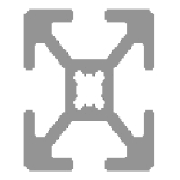
# Autodesk Inventor part: 20-2020
Saved by Autodesk Inventor 2021 (Build 250183000, 183)
## iProperties
Created: 2020-11-08
Part Number: 20-2020
Material: Generic
Document SubType Name: Modeling
Designer: Wes
Manufacturer: 8020
Standards Organization: 8020 Metric
Language: en-US
Size Designation: 20-2020
Categories: <MemberInstance><Categories><Category DisplayName="Structural Shapes" InternalName="089c4875-fa83-4c05-b084-43b9cc11f5ed" Mnemonic="GRDR"><CategoryParameter DisplayName="Mass per Length Unit" InternalName="0bb95a10-148f-4027-a459-38d7b056702a" Mnemonic="shpmass"/><CategoryParameter DisplayName="Section Area" InternalName="1ff91680-64b0-4202-b9a3-7fd3f94bba3b" Mnemonic="secarea"/><CategoryParameter DisplayName="Radius of Gyration (x)" InternalName="25778675-03e9-40c1-b6a8-4a9ed693320d" Mnemonic="gyrradx"/><CategoryParameter DisplayName="Torsional Rigidity Modulus" InternalName="26c1ec35-5026-4c63-ad0a-751cf684a536" Mnemonic="torrigmod"/><CategoryParameter DisplayName="Distance of the Center of Gravity X-X" InternalName="26c9bdb8-9c79-4b4f-a92e-8e197583c9c4" Mnemonic="grcendistX"/><CategoryParameter DisplayName="Legacy Member ID" InternalName="340afe4f-75d7-48d3-ab7d-943f3c3da468" Mnemonic="LegacyMemberID"/><CategoryParameter DisplayName="Base Length" InternalName="42e34263-8f20-4d0e-ad48-bf1385b87c24" Mnemonic="shplen"/><CategoryParameter DisplayName="Moment of Inertia (y)" InternalName="4b9f58ea-bced-460e-81ea-3d29ca5a49e3" Mnemonic="inermomy"/><CategoryParameter DisplayName="Moment of Inertia (x)" InternalName="4cd780bc-73d7-43ac-917a-579e5cbd684d" Mnemonic="inermomx"/><CategoryParameter DisplayName="Custom Base Point" InternalName="4f1d1b73-316d-484b-a3df-9cbabb16eb77" Mnemonic="shpBasePoint"/><CategoryParameter DisplayName="Shape Height" InternalName="50274e7d-5ac0-4796-92cb-c59e54983c67" Mnemonic="shpheig"/><CategoryParameter DisplayName="Section Module (y)" InternalName="59eaa5e9-d227-48dc-b6c1-6920f96e0f95" Mnemonic="secmody"/><CategoryParameter DisplayName="Section Designation" InternalName="5a64d034-428d-49c8-ba32-7619764de20f" Mnemonic="shpdes"/><CategoryParameter DisplayName="Section Module (x)" InternalName="72cfad18-cf51-4ed4-aaa7-c6b224f8419f" Mnemonic="secmodx"/><CategoryParameter DisplayName="Torsional Section Modulus" InternalName="7c55a8dc-8844-49f9-a867-cc677b30ec9a" Mnemonic="torsecmod"/><CategoryParameter DisplayName="Shape Width" InternalName="7c717d54-a18f-4666-b4d4-573cce22c62c" Mnemonic="shpwdth"/><CategoryParameter DisplayName="Second Shape Thickness" InternalName="9251a8e1-85fd-4e47-af99-afdb762317d9" Mnemonic="shpthick2"/><CategoryParameter DisplayName="FG Authored" InternalName="9c666724-f362-4ea7-ac62-f6a007de5c69" Mnemonic="shpFGAuto"/><CategoryParameter DisplayName="Distance of the Center of Gravity Y-Y" InternalName="bcc4fb17-7af4-436a-8f8c-d0aa3b0248c5" Mnemonic="grcendistY"/><CategoryParameter DisplayName="Radius of Gyration (y)" InternalName="bfa18ebe-1636-4dbe-8d42-b263e0b73184" Mnemonic="gyrrady"/><CategoryParameter DisplayName="Shape Thickness" InternalName="d109cf76-8eb4-42fc-9800-4409734adc67" Mnemonic="shpthick"/><CategoryParameter DisplayName="Coefficient of Shear Displacement" InternalName="de4c90c6-aaa8-468f-a335-6737b311b5d3" Mnemonic="shdispc"/><Category DisplayName="Other" InternalName="f02205ff-2390-476f-921c-0b3185f88e84" Mnemonic="OTHSHP"><CategoryParameter DisplayName="Moment of Inertia (y)" InternalName="044c654e-f649-48ac-84cc-650a29ae31ca" Mnemonic="inermomy"/><CategoryParameter DisplayName="Shape Thickness" InternalName="12b1a788-9233-48fd-a933-2df8ff42b15f" Mnemonic="shpthick"/><CategoryParameter DisplayName="Mass per Length Unit" InternalName="2fd289d6-9394-4d2d-97e6-6659d7d4551d" Mnemonic="shpmass"/><CategoryParameter DisplayName="Radius of Gyration (y)" InternalName="743e1dfe-1bba-408b-b985-cf752b207386" Mnemonic="gyrrady"/><CategoryParameter DisplayName="Section Module (y)" InternalName="88b8bff9-a616-4028-93d5-ed4f79680d13" Mnemonic="secmody"/><CategoryParameter DisplayName="Section Area" InternalName="c46ecdf8-b6eb-4db9-8b25-30258930c1e3" Mnemonic="secarea"/><CategoryParameter DisplayName="Section Module (x)" InternalName="cac70804-9d39-43bb-be17-56ea1f39a6c2" Mnemonic="secmodx"/><CategoryParameter DisplayName="Moment of Inertia (x)" InternalName="ec6737bc-264f-43ed-b0bd-f6d410c2718d" Mnemonic="inermomx"/><CategoryParameter DisplayName="Radius of Gyration (x)" InternalName="ee72c61e-565e-4fd6-b448-66e1e1abcb7e" Mnemonic="gyrradx"/><Category DisplayName="8020" InternalName="79851eee-1260-43d5-80eb-d25638456875" Mnemonic="8020"/></Category></Category><Category DisplayName="DataType" InternalName="23b78d0f-2648-40c6-8793-ca6db495c9e8" Mnemonic="DATATYPE"><CategoryParameter DisplayName="DisplayName" InternalName="05415f3d-3907-474b-a020-eb9d644f4cf3" Mnemonic="DISPLAYNAME"/><CategoryParameter DisplayName="Standard" InternalName="0c0a119c-1e12-4c84-803f-101930972f5e" Mnemonic="STANDARD"/><CategoryParameter DisplayName="Description" InternalName="13903e3d-64b1-4950-80da-f627842ea37f" Mnemonic="DESCRIPTION"/><CategoryParameter DisplayName="Designation" InternalName="2675968c-4ce5-49e0-a4f5-552d29089031" Mnemonic="DESIGNATION"/><CategoryParameter DisplayName="Default Row" InternalName="2af9ec52-faaa-4026-b378-f9fa4afca842" Mnemonic="DEFAULTROW"/><CategoryParameter DisplayName="Folder Name" InternalName="3f06958e-8713-4116-9be7-ed6184ecc97b" Mnemonic="FOLDERNAME"/><CategoryParameter DisplayName="Revision Guid" InternalName="45a75005-10b1-4dfc-8d6d-dfe629f0b93c" Mnemonic="REVISIONGUID"/><CategoryParameter DisplayName="FileName" InternalName="8b46a4cc-9585-4fed-90c3-899f57e09a73" Mnemonic="FILENAME"/><CategoryParameter DisplayName="StdsOrg" InternalName="8f5914e1-4693-403f-8ab5-d37768198c9d" Mnemonic="STDSORG"/><CategoryParameter DisplayName="Family Version" InternalName="914462f6-6e19-4b14-ba84-155b9680b1d0" Mnemonic="FAMILYREVISION"/><CategoryParameter DisplayName="Standard Revision" InternalName="91d5a463-65c2-4fde-b823-3b7fea5e8e17" Mnemonic="STANDARDREVISION"/><CategoryParameter DisplayName="Member Revision" InternalName="a65d44b9-392f-4f4f-857b-e4b3d54996fe" Mnemonic="MEMBERREVISION"/><CategoryParameter DisplayName="ClipFormat" InternalName="bc51e27b-3422-4e78-93ef-cec197ddf230" Mnemonic="CLIPFORMAT"/><CategoryParameter DisplayName="Manufacturer" InternalName="cd6c7a72-a28a-4e50-99a9-2c7f4e13e5ad" Mnemonic="MANUFACTURER"/><CategoryParameter DisplayName="InternalName" InternalName="cf1d0246-76d9-4b4a-8305-fa0409afb5c1" Mnemonic="INTERNALNAME"/><CategoryParameter DisplayName="IsMetric" InternalName="e2385c5b-1ea4-4823-96a8-8de651266ec3" Mnemonic="ISMETRIC"/><Category DisplayName="Part" InternalName="c0e0b642-3bcb-4cc8-9e80-f96d35c4afa4" Mnemonic="PART"><CategoryParameter DisplayName="Part Number" InternalName="016b6077-bfbe-49bd-92c9-d8d59c39c941" Mnemonic="PARTNUMBER"/><CategoryParameter DisplayName="Stock Number" InternalName="4dba7c1c-e26c-444e-836c-b08b433409a8" Mnemonic="STOCKNUMBER"/><CategoryParameter DisplayName="Material Key" InternalName="5c9a8adb-dd2b-4535-b97f-0a94a95fe41f" Mnemonic="MATERIALKEY"/><CategoryParameter DisplayName="Material" InternalName="818a152a-d3c3-49ca-80ee-df7d91421b8e" Mnemonic="MATERIAL"/></Category></Category></Categories><FamilyTemplate Id="20-2020"><FamilyTemplateParameters><FamilyTemplateParameter ObjectType="kModelParameterObject" ValueType="xs:double" Id="12" ObjectReferenceKey="Length"/><FamilyTemplateParameter ObjectType="kPartComponentDefinitionObject" ValueType="xs:string" Id="23" SubObjectId="Material"/><FamilyTemplateParameter ObjectType="kPropertyObject" ValueType="xs:string" Id="26" ObjectReferenceKey="{32853F0F-3444-11d1-9E93-0060B03C1CA6}" SubObjectId="5"/><FamilyTemplateParameter ObjectType="kPropertyObject" ValueType="xs:string" Id="27" ObjectReferenceKey="{32853F0F-3444-11d1-9E93-0060B03C1CA6}" SubObjectId="52"/></FamilyTemplateParameters></FamilyTemplate><CategoryParameterMap><ParamToTemplateMap><ParamToTemplate CategoryParameter="//CategoryParameter[@InternalName='cf1d0246-76d9-4b4a-8305-fa0409afb5c1']" ConstantValue="c23acc55-1e46-463f-aee6-b755883656a5"/><ParamToTemplate CategoryParameter="//CategoryParameter[@InternalName='45a75005-10b1-4dfc-8d6d-dfe629f0b93c']" ConstantValue="7ed192ba-9534-4655-9213-06d96e12c78c"/><ParamToTemplate CategoryParameter="//CategoryParameter[@InternalName='3f06958e-8713-4116-9be7-ed6184ecc97b']" ConstantValue="20-2020"/><ParamToTemplate CategoryParameter="//CategoryParameter[@InternalName='8f5914e1-4693-403f-8ab5-d37768198c9d']" ConstantValue="8020 Metric"/><ParamToTemplate CategoryParameter="//CategoryParameter[@InternalName='0c0a119c-1e12-4c84-803f-101930972f5e']" TemplateParameter="18"/><ParamToTemplate CategoryParameter="//CategoryParameter[@InternalName='91d5a463-65c2-4fde-b823-3b7fea5e8e17']" TemplateParameter="19"/><ParamToTemplate CategoryParameter="//CategoryParameter[@InternalName='cd6c7a72-a28a-4e50-99a9-2c7f4e13e5ad']" ConstantValue="8020"/><ParamToTemplate CategoryParameter="//CategoryParameter[@InternalName='13903e3d-64b1-4950-80da-f627842ea37f']" TemplateParameter="22"/><ParamToTemplate CategoryParameter="//CategoryParameter[@InternalName='05415f3d-3907-474b-a020-eb9d644f4cf3']" ConstantValue="20-2020"/><ParamToTemplate CategoryParameter="//CategoryParameter[@InternalName='914462f6-6e19-4b14-ba84-155b9680b1d0']" ConstantValue="11"/><ParamToTemplate CategoryParameter="//CategoryParameter[@InternalName='bc51e27b-3422-4e78-93ef-cec197ddf230']" ConstantValue="CF_INVENTOR.STDPARTS"/><ParamToTemplate CategoryParameter="//CategoryParameter[@InternalName='e2385c5b-1ea4-4823-96a8-8de651266ec3']" ConstantValue="false"/><ParamToTemplate CategoryParameter="//CategoryParameter[@InternalName='2af9ec52-faaa-4026-b378-f9fa4afca842']" ConstantValue="1"/><ParamToTemplate CategoryParameter="//CategoryParameter[@InternalName='9c666724-f362-4ea7-ac62-f6a007de5c69']" ConstantValue="1"/><ParamToTemplate CategoryParameter="//CategoryParameter[@InternalName='8b46a4cc-9585-4fed-90c3-899f57e09a73']" ConstantValue="20-2020"/><ParamToTemplate CategoryParameter="//CategoryParameter[@InternalName='a65d44b9-392f-4f4f-857b-e4b3d54996fe']" ConstantValue="fbe24d84-f0ed-4629-ad88-4417b9aca3a2"/><ParamToTemplate CategoryParameter="//CategoryParameter[@InternalName='a65d44b9-392f-4f4f-857b-e4b3d54996fe']" ConstantValue="fbe24d84-f0ed-4629-ad88-4417b9aca3a2"/><ParamToTemplate CategoryParameter="//CategoryParameter[@InternalName='2675968c-4ce5-49e0-a4f5-552d29089031']" TemplateParameter="27"/><ParamToTemplate CategoryParameter="//CategoryParameter[@InternalName='42e34263-8f20-4d0e-ad48-bf1385b87c24']" TemplateParameter="12"/><ParamToTemplate CategoryParameter="//CategoryParameter[@InternalName='818a152a-d3c3-49ca-80ee-df7d91421b8e']" TemplateParameter="23"/><ParamToTemplate CategoryParameter="//CategoryParameter[@InternalName='016b6077-bfbe-49bd-92c9-d8d59c39c941']" TemplateParameter="26"/></ParamToTemplateMap></CategoryParameterMap></MemberInstance>
Density: 1 g/cm^3
Appearance: Default
IsCustomPart: 1
_CCFamilyDisplayName: 20-2020
_FrameMemberDoc: Frame Member File
_Version: 15.0.0
_GetPNFromCC: 1
Author: Wes
G_L: 32.165 in
G_W: 0.787 in
G_H: 0.787 in
+A867D917-BCFB-4BDE-AF9A-2008976AA419+CUTDETAIL1: Cut Angle 90.00 deg
Autodesk Inventor part; units mm, degrees
ref_plane "YZ Plane" through (0, 0, 0) normal (1, 0, 0) x (0, 1, 0)
ref_plane "XZ Plane" through (0, 0, 0) normal (0, 1, 0) x (-1, 0, 0)
sketch "20-2020" plane through (0, 0, 0) normal (0, 0, 1) x (1, 0, 0)
  arc A0 (19.287, 13.8034) -> (20.6079, 13.434) centre (20.0514, 13.9905) ccw
  line L0 (20.6079, 13.434) -> (20.7875, 13.6136)
  arc A1 (20.7875, 13.6136) -> (20.4182, 14.9345) centre (20.231, 14.1701) ccw
  arc A2 (20.4182, 14.9345) -> (20.4182, 16.5425) centre (18.483, 15.7385) ccw
  arc A3 (20.4182, 16.5425) -> (20.7875, 17.8634) centre (20.231, 17.3069) ccw
  line L1 (20.7875, 17.8634) -> (20.6079, 18.043)
  arc A4 (20.6079, 18.043) -> (19.287, 17.6736) centre (20.0514, 17.4865) ccw
  arc A5 (19.287, 17.6736) -> (17.679, 17.6736) centre (18.483, 15.7385) ccw
  arc A6 (17.679, 17.6736) -> (16.3581, 18.043) centre (16.9146, 17.4865) ccw
  line L2 (16.3581, 18.043) -> (16.1785, 17.8634)
  arc A7 (16.1785, 17.8634) -> (16.5479, 16.5425) centre (16.735, 17.3069) ccw
  arc A8 (16.5479, 16.5425) -> (16.5479, 14.9345) centre (18.483, 15.7385) ccw
  arc A9 (16.5479, 14.9345) -> (16.1785, 13.6136) centre (16.735, 14.1701) ccw
  line L3 (16.1785, 13.6136) -> (16.3581, 13.434)
  arc A10 (16.3581, 13.434) -> (17.679, 13.8034) centre (16.9146, 13.9905) ccw
  arc A11 (17.679, 13.8034) -> (19.287, 13.8034) centre (18.483, 15.7385) ccw
  line L4 (27.491, 18.3685) -> (27.975, 18.3685)
  arc A12 (26.983, 18.8765) -> (27.491, 18.3685) centre (27.491, 18.8765) ccw
  line L5 (26.983, 21.2255) -> (26.983, 18.8765)
  arc A13 (26.983, 21.2255) -> (26.475, 21.7335) centre (26.475, 21.2255) ccw
  line L6 (25.7491, 21.7335) -> (26.475, 21.7335)
  arc A14 (25.7491, 21.7335) -> (25.3899, 21.5847) centre (25.7491, 21.2255) ccw
  line L7 (22.2868, 18.4816) -> (25.3899, 21.5847)
  arc A15 (22.2868, 18.4816) -> (22.138, 18.1224) centre (22.646, 18.1224) ccw
  line L8 (22.138, 13.3546) -> (22.138, 18.1224)
  arc A16 (22.138, 13.3546) -> (22.2868, 12.9954) centre (22.646, 13.3546) ccw
  line L9 (25.3899, 9.8923) -> (22.2868, 12.9954)
  arc A17 (25.3899, 9.8923) -> (25.7491, 9.7435) centre (25.7491, 10.2515) ccw
  line L10 (26.475, 9.7435) -> (25.7491, 9.7435)
  arc A18 (26.475, 9.7435) -> (26.983, 10.2515) centre (26.475, 10.2515) ccw
  line L11 (26.983, 12.6005) -> (26.983, 10.2515)
  arc A19 (27.491, 13.1085) -> (26.983, 12.6005) centre (27.491, 12.6005) ccw
  line L12 (27.975, 13.1085) -> (27.491, 13.1085)
  arc A20 (28.483, 12.6005) -> (27.975, 13.1085) centre (27.975, 12.6005) ccw
  line L13 (28.483, 7.2385) -> (28.483, 12.6005)
  arc A21 (26.983, 5.7385) -> (28.483, 7.2385) centre (26.983, 7.2385) ccw
  line L14 (21.621, 5.7385) -> (26.983, 5.7385)
  arc A22 (21.113, 6.2465) -> (21.621, 5.7385) centre (21.621, 6.2465) ccw
  line L15 (21.113, 6.7305) -> (21.113, 6.2465)
  arc A23 (21.621, 7.2385) -> (21.113, 6.7305) centre (21.621, 6.7305) ccw
  line L16 (23.97, 7.2385) -> (21.621, 7.2385)
  arc A24 (23.97, 7.2385) -> (24.478, 7.7465) centre (23.97, 7.7465) ccw
  line L17 (24.478, 8.4724) -> (24.478, 7.7465)
  arc A25 (24.478, 8.4724) -> (24.3292, 8.8316) centre (23.97, 8.4724) ccw
  line L18 (21.2261, 11.9347) -> (24.3292, 8.8316)
  arc A26 (21.2261, 11.9347) -> (20.8669, 12.0835) centre (20.8669, 11.5755) ccw
  line L19 (16.0991, 12.0835) -> (20.8669, 12.0835)
  arc A27 (16.0991, 12.0835) -> (15.7399, 11.9347) centre (16.0991, 11.5755) ccw
  line L20 (12.6368, 8.8316) -> (15.7399, 11.9347)
  arc A28 (12.6368, 8.8316) -> (12.488, 8.4724) centre (12.996, 8.4724) ccw
  line L21 (12.488, 7.7465) -> (12.488, 8.4724)
  arc A29 (12.488, 7.7465) -> (12.996, 7.2385) centre (12.996, 7.7465) ccw
  line L22 (15.345, 7.2385) -> (12.996, 7.2385)
  arc A30 (15.853, 6.7305) -> (15.345, 7.2385) centre (15.345, 6.7305) ccw
  line L23 (15.853, 6.2465) -> (15.853, 6.7305)
  arc A31 (15.345, 5.7385) -> (15.853, 6.2465) centre (15.345, 6.2465) ccw
  line L24 (9.983, 5.7385) -> (15.345, 5.7385)
  arc A32 (8.483, 7.2385) -> (9.983, 5.7385) centre (9.983, 7.2385) ccw
  line L25 (8.483, 12.6005) -> (8.483, 7.2385)
  arc A33 (8.991, 13.1085) -> (8.483, 12.6005) centre (8.991, 12.6005) ccw
  line L26 (9.475, 13.1085) -> (8.991, 13.1085)
  arc A34 (9.983, 12.6005) -> (9.475, 13.1085) centre (9.475, 12.6005) ccw
  line L27 (9.983, 10.2515) -> (9.983, 12.6005)
  arc A35 (9.983, 10.2515) -> (10.491, 9.7435) centre (10.491, 10.2515) ccw
  line L28 (11.2169, 9.7435) -> (10.491, 9.7435)
  arc A36 (11.2169, 9.7435) -> (11.5761, 9.8923) centre (11.2169, 10.2515) ccw
  line L29 (14.6792, 12.9954) -> (11.5761, 9.8923)
  arc A37 (14.6792, 12.9954) -> (14.828, 13.3546) centre (14.32, 13.3546) ccw
  line L30 (14.828, 18.1224) -> (14.828, 13.3546)
  arc A38 (14.828, 18.1224) -> (14.6792, 18.4816) centre (14.32, 18.1224) ccw
  line L31 (11.5761, 21.5847) -> (14.6792, 18.4816)
  arc A39 (11.5761, 21.5847) -> (11.2169, 21.7335) centre (11.2169, 21.2255) ccw
  line L32 (10.491, 21.7335) -> (11.2169, 21.7335)
  arc A40 (10.491, 21.7335) -> (9.983, 21.2255) centre (10.491, 21.2255) ccw
  line L33 (9.983, 18.8765) -> (9.983, 21.2255)
  arc A41 (9.475, 18.3685) -> (9.983, 18.8765) centre (9.475, 18.8765) ccw
  line L34 (8.991, 18.3685) -> (9.475, 18.3685)
  arc A42 (8.483, 18.8765) -> (8.991, 18.3685) centre (8.991, 18.8765) ccw
  line L35 (8.483, 24.2385) -> (8.483, 18.8765)
  arc A43 (9.983, 25.7385) -> (8.483, 24.2385) centre (9.983, 24.2385) ccw
  line L36 (15.345, 25.7385) -> (9.983, 25.7385)
  arc A44 (15.853, 25.2305) -> (15.345, 25.7385) centre (15.345, 25.2305) ccw
  line L37 (15.853, 24.7465) -> (15.853, 25.2305)
  arc A45 (15.345, 24.2385) -> (15.853, 24.7465) centre (15.345, 24.7465) ccw
  line L38 (12.996, 24.2385) -> (15.345, 24.2385)
  arc A46 (12.996, 24.2385) -> (12.488, 23.7305) centre (12.996, 23.7305) ccw
  line L39 (12.488, 23.0046) -> (12.488, 23.7305)
  arc A47 (12.488, 23.0046) -> (12.6368, 22.6454) centre (12.996, 23.0046) ccw
  line L40 (15.7399, 19.5423) -> (12.6368, 22.6454)
  arc A48 (15.7399, 19.5423) -> (16.0991, 19.3935) centre (16.0991, 19.9015) ccw
  line L41 (20.8669, 19.3935) -> (16.0991, 19.3935)
  arc A49 (20.8669, 19.3935) -> (21.2261, 19.5423) centre (20.8669, 19.9015) ccw
  line L42 (24.3292, 22.6454) -> (21.2261, 19.5423)
  arc A50 (24.3292, 22.6454) -> (24.478, 23.0046) centre (23.97, 23.0046) ccw
  line L43 (24.478, 23.7305) -> (24.478, 23.0046)
  arc A51 (24.478, 23.7305) -> (23.97, 24.2385) centre (23.97, 23.7305) ccw
  line L44 (21.621, 24.2385) -> (23.97, 24.2385)
  arc A52 (21.113, 24.7465) -> (21.621, 24.2385) centre (21.621, 24.7465) ccw
  line L45 (21.113, 25.2305) -> (21.113, 24.7465)
  arc A53 (21.621, 25.7385) -> (21.113, 25.2305) centre (21.621, 25.2305) ccw
  line L46 (26.983, 25.7385) -> (21.621, 25.7385)
  arc A54 (28.483, 24.2385) -> (26.983, 25.7385) centre (26.983, 24.2385) ccw
  line L47 (28.483, 18.8765) -> (28.483, 24.2385)
  arc A55 (27.975, 18.3685) -> (28.483, 18.8765) centre (27.975, 18.8765) ccw
ref_plane "Start Plane" through (0, 0, 20) normal (0, 0, 1) x (1, 0, 0)
ref_plane "End Plane" through (0, 0, 837) normal (0, 0, 1) x (1, 0, 0)
sketch "Sketch" plane through (0, 0, 0) normal (0, 0, 1) x (1, 0, 0)
  arc A0 (0.804, -1.9351) -> (2.1249, -2.3045) centre (1.5684, -1.748) ccw
  line L0 (2.1249, -2.3045) -> (2.3045, -2.1249)
  arc A1 (2.3045, -2.1249) -> (1.9351, -0.804) centre (1.748, -1.5684) ccw
  arc A2 (1.9351, -0.804) -> (1.9351, 0.804) centre (0, 0) ccw
  arc A3 (1.9351, 0.804) -> (2.3045, 2.1249) centre (1.748, 1.5684) ccw
  line L1 (2.3045, 2.1249) -> (2.1249, 2.3045)
  arc A4 (2.1249, 2.3045) -> (0.804, 1.9351) centre (1.5684, 1.748) ccw
  arc A5 (0.804, 1.9351) -> (-0.804, 1.9351) centre (0, 0) ccw
  arc A6 (-0.804, 1.9351) -> (-2.1249, 2.3045) centre (-1.5684, 1.748) ccw
  line L2 (-2.1249, 2.3045) -> (-2.3045, 2.1249)
  arc A7 (-2.3045, 2.1249) -> (-1.9351, 0.804) centre (-1.748, 1.5684) ccw
  arc A8 (-1.9351, 0.804) -> (-1.9351, -0.804) centre (0, 0) ccw
  arc A9 (-1.9351, -0.804) -> (-2.3045, -2.1249) centre (-1.748, -1.5684) ccw
  line L3 (-2.3045, -2.1249) -> (-2.1249, -2.3045)
  arc A10 (-2.1249, -2.3045) -> (-0.804, -1.9351) centre (-1.5684, -1.748) ccw
  arc A11 (-0.804, -1.9351) -> (0.804, -1.9351) centre (0, 0) ccw
  line L4 (9.008, 2.63) -> (9.492, 2.63)
  arc A12 (8.5, 3.138) -> (9.008, 2.63) centre (9.008, 3.138) ccw
  line L5 (8.5, 5.487) -> (8.5, 3.138)
  arc A13 (8.5, 5.487) -> (7.992, 5.995) centre (7.992, 5.487) ccw
  line L6 (7.2661, 5.995) -> (7.992, 5.995)
  arc A14 (7.2661, 5.995) -> (6.9069, 5.8462) centre (7.2661, 5.487) ccw
  line L7 (3.8038, 2.7431) -> (6.9069, 5.8462)
  arc A15 (3.8038, 2.7431) -> (3.655, 2.3839) centre (4.163, 2.3839) ccw
  line L8 (3.655, -2.3839) -> (3.655, 2.3839)
  arc A16 (3.655, -2.3839) -> (3.8038, -2.7431) centre (4.163, -2.3839) ccw
  line L9 (6.9069, -5.8462) -> (3.8038, -2.7431)
  arc A17 (6.9069, -5.8462) -> (7.2661, -5.995) centre (7.2661, -5.487) ccw
  line L10 (7.992, -5.995) -> (7.2661, -5.995)
  arc A18 (7.992, -5.995) -> (8.5, -5.487) centre (7.992, -5.487) ccw
  line L11 (8.5, -3.138) -> (8.5, -5.487)
  arc A19 (9.008, -2.63) -> (8.5, -3.138) centre (9.008, -3.138) ccw
  line L12 (9.492, -2.63) -> (9.008, -2.63)
  arc A20 (10, -3.138) -> (9.492, -2.63) centre (9.492, -3.138) ccw
  line L13 (10, -8.5) -> (10, -3.138)
  arc A21 (8.5, -10) -> (10, -8.5) centre (8.5, -8.5) ccw
  line L14 (3.138, -10) -> (8.5, -10)
  arc A22 (2.63, -9.492) -> (3.138, -10) centre (3.138, -9.492) ccw
  line L15 (2.63, -9.008) -> (2.63, -9.492)
  arc A23 (3.138, -8.5) -> (2.63, -9.008) centre (3.138, -9.008) ccw
  line L16 (5.487, -8.5) -> (3.138, -8.5)
  arc A24 (5.487, -8.5) -> (5.995, -7.992) centre (5.487, -7.992) ccw
  line L17 (5.995, -7.2661) -> (5.995, -7.992)
  arc A25 (5.995, -7.2661) -> (5.8462, -6.9069) centre (5.487, -7.2661) ccw
  line L18 (2.7431, -3.8038) -> (5.8462, -6.9069)
  arc A26 (2.7431, -3.8038) -> (2.3839, -3.655) centre (2.3839, -4.163) ccw
  line L19 (-2.3839, -3.655) -> (2.3839, -3.655)
  arc A27 (-2.3839, -3.655) -> (-2.7431, -3.8038) centre (-2.3839, -4.163) ccw
  line L20 (-5.8462, -6.9069) -> (-2.7431, -3.8038)
  arc A28 (-5.8462, -6.9069) -> (-5.995, -7.2661) centre (-5.487, -7.2661) ccw
  line L21 (-5.995, -7.992) -> (-5.995, -7.2661)
  arc A29 (-5.995, -7.992) -> (-5.487, -8.5) centre (-5.487, -7.992) ccw
  line L22 (-3.138, -8.5) -> (-5.487, -8.5)
  arc A30 (-2.63, -9.008) -> (-3.138, -8.5) centre (-3.138, -9.008) ccw
  line L23 (-2.63, -9.492) -> (-2.63, -9.008)
  arc A31 (-3.138, -10) -> (-2.63, -9.492) centre (-3.138, -9.492) ccw
  line L24 (-8.5, -10) -> (-3.138, -10)
  arc A32 (-10, -8.5) -> (-8.5, -10) centre (-8.5, -8.5) ccw
  line L25 (-10, -3.138) -> (-10, -8.5)
  arc A33 (-9.492, -2.63) -> (-10, -3.138) centre (-9.492, -3.138) ccw
  line L26 (-9.008, -2.63) -> (-9.492, -2.63)
  arc A34 (-8.5, -3.138) -> (-9.008, -2.63) centre (-9.008, -3.138) ccw
  line L27 (-8.5, -5.487) -> (-8.5, -3.138)
  arc A35 (-8.5, -5.487) -> (-7.992, -5.995) centre (-7.992, -5.487) ccw
  line L28 (-7.2661, -5.995) -> (-7.992, -5.995)
  arc A36 (-7.2661, -5.995) -> (-6.9069, -5.8462) centre (-7.2661, -5.487) ccw
  line L29 (-3.8038, -2.7431) -> (-6.9069, -5.8462)
  arc A37 (-3.8038, -2.7431) -> (-3.655, -2.3839) centre (-4.163, -2.3839) ccw
  line L30 (-3.655, 2.3839) -> (-3.655, -2.3839)
  arc A38 (-3.655, 2.3839) -> (-3.8038, 2.7431) centre (-4.163, 2.3839) ccw
  line L31 (-6.9069, 5.8462) -> (-3.8038, 2.7431)
  arc A39 (-6.9069, 5.8462) -> (-7.2661, 5.995) centre (-7.2661, 5.487) ccw
  line L32 (-7.992, 5.995) -> (-7.2661, 5.995)
  arc A40 (-7.992, 5.995) -> (-8.5, 5.487) centre (-7.992, 5.487) ccw
  line L33 (-8.5, 3.138) -> (-8.5, 5.487)
  arc A41 (-9.008, 2.63) -> (-8.5, 3.138) centre (-9.008, 3.138) ccw
  line L34 (-9.492, 2.63) -> (-9.008, 2.63)
  arc A42 (-10, 3.138) -> (-9.492, 2.63) centre (-9.492, 3.138) ccw
  line L35 (-10, 8.5) -> (-10, 3.138)
  arc A43 (-8.5, 10) -> (-10, 8.5) centre (-8.5, 8.5) ccw
  line L36 (-3.138, 10) -> (-8.5, 10)
  arc A44 (-2.63, 9.492) -> (-3.138, 10) centre (-3.138, 9.492) ccw
  line L37 (-2.63, 9.008) -> (-2.63, 9.492)
  arc A45 (-3.138, 8.5) -> (-2.63, 9.008) centre (-3.138, 9.008) ccw
  line L38 (-5.487, 8.5) -> (-3.138, 8.5)
  arc A46 (-5.487, 8.5) -> (-5.995, 7.992) centre (-5.487, 7.992) ccw
  line L39 (-5.995, 7.2661) -> (-5.995, 7.992)
  arc A47 (-5.995, 7.2661) -> (-5.8462, 6.9069) centre (-5.487, 7.2661) ccw
  line L40 (-2.7431, 3.8038) -> (-5.8462, 6.9069)
  arc A48 (-2.7431, 3.8038) -> (-2.3839, 3.655) centre (-2.3839, 4.163) ccw
  line L41 (2.3839, 3.655) -> (-2.3839, 3.655)
  arc A49 (2.3839, 3.655) -> (2.7431, 3.8038) centre (2.3839, 4.163) ccw
  line L42 (5.8462, 6.9069) -> (2.7431, 3.8038)
  arc A50 (5.8462, 6.9069) -> (5.995, 7.2661) centre (5.487, 7.2661) ccw
  line L43 (5.995, 7.992) -> (5.995, 7.2661)
  arc A51 (5.995, 7.992) -> (5.487, 8.5) centre (5.487, 7.992) ccw
  line L44 (3.138, 8.5) -> (5.487, 8.5)
  arc A52 (2.63, 9.008) -> (3.138, 8.5) centre (3.138, 9.008) ccw
  line L45 (2.63, 9.492) -> (2.63, 9.008)
  arc A53 (3.138, 10) -> (2.63, 9.492) centre (3.138, 9.492) ccw
  line L46 (8.5, 10) -> (3.138, 10)
  arc A54 (10, 8.5) -> (8.5, 10) centre (8.5, 8.5) ccw
  line L47 (10, 3.138) -> (10, 8.5)
  arc A55 (9.492, 2.63) -> (10, 3.138) centre (9.492, 3.138) ccw
  point P0 (0, 0)
  constraints: 1 other
extrude "Body" add sketch "Sketch" along normal up to surface (817 mm away) from surface at 20
sketch "Sketch2" plane through (0, 0, 0) normal (0, 0, 1) x (1, 0, 0)
  line L0 (0, 0) -> (10, 0)
ref_plane "Work Plane3" through (0, 0, 0) normal (0, -1, 0) x (1, 0, 0)
sketch "Sketch3" plane through (0, 0, 0) normal (0, -1, 0) x (1, 0, 0)
  line L0 (-2, 20) -> (12, 20)
  line L1 (-2, 837) -> (12, 837)
  dimension "d7" = 817
  measures "d7" distance between parallel lines of L0 L1
ref_plane "Work Plane4" through (-827, 8.5, 20) normal (0, 0, -1) x (-1, 0, 0)
split "Split1" plane through (-827, 8.5, 20) removes the side toward (0, 0, -1)
equation "\"G_OFFSET_START\" = -20"
equation "\"G_OFFSET_END\" = 0"
equation "\"d2\" = -G_OFFSET_START"
equation "\"d3\" = Length + G_OFFSET_END"
equation "\"G_L\" = d7"
equation "\"Length\" = 837"
body "Solid1"
